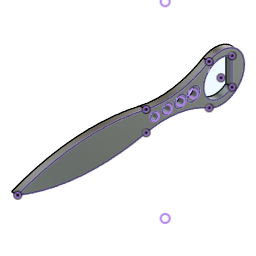
OpenBottleOpener (Autodesk Fusion 360 design; units mm, degrees)
Autodesk Fusion 360 part; units mm, degrees
sketch "Shape" plane through (0, 0, 0) normal (1, 0, 0) x (0, 1, 0)
  arc A0 (99.06, 7.7917) -> (0, 0) centre (62.0114, -154.7864) ccw
  arc A1 (99.06, 7.7917) -> (147.7109, 15.4666) centre (113.7922, 72.4404) ccw
  arc A2 (174.9187, 0) -> (147.7109, 15.4666) centre (156.9187, 0) ccw
  line L0 (0, 0) -> (174.9187, 0)
  arc A3 (170.4187, 0) -> (143.4187, 0) centre (156.9187, 0) ccw
  line L1 (165.4187, 10.4881) -> (165.4187, 0)
  circle A4 centre (115.4187, 0) radius 3.6667
  circle A5 centre (125.4187, 0) radius 4.3333
  circle A6 centre (135.4187, 0) radius 5
  circle A7 centre (105.4187, 0) radius 3
  line L2 (105.2187, -2.9933) -> (135.0854, -4.9889)
  line L3 (105.4187, 0) -> (115.4187, 0)
  line L4 (115.4187, 0) -> (125.4187, 0)
  line L5 (125.4187, 0) -> (135.4187, 0)
  line L6 (102.4187, 0) -> (0, 0)
  line L7 (140.4187, 0) -> (143.4187, 0)
  line L8 (170.4187, 0) -> (174.9187, 0)
  line L9 (170.4187, 0) -> (165.4187, 0)
  dimension "d2" = 99.06
  dimension "d3" = 18
  dimension "d10" = 174.9187
  dimension "d11" = 13.5
  dimension "d12" = 8.5
  dimension "d13" = 6
  dimension "d14" = 10
  dimension "d15" = 10
  dimension "d16" = 8
  constraint coincident A0.end L0.start
  constraint horizontal L0
  constraint tangent A0 A1
  constraint tangent A1 A2
  constraint horizontal A2.start A2.centre
  constraint coincident L0 A3.start
  constraint coincident A2.centre A3.centre
  constraint coincident L0 A3.end
  constraint coincident A3 L1.start
  constraint coincident L0 L1.end
  constraint perpendicular L0 L1
  constraint coincident L0 A4.centre
  constraint coincident L0 A5.centre
  constraint coincident L0 A6.centre
  constraint coincident L0 A7.centre
  constraint coincident A7 L2.start
  constraint coincident A6 L2.end
  constraint tangent A6 L2
  constraint tangent A7 L2
  constraint tangent A5 L2
  constraint tangent A4 L2
  constraint coincident A7.centre L3.start
  constraint coincident A4.centre L3.end
  constraint coincident A5.centre L4.end
  constraint coincident A6.centre L5.end
  constraint equal L3 L4
  constraint equal L4 L5
  constraint coincident A7 L6.start
  constraint coincident L0 L6.start
  constraint coincident A6 L7.start
  constraint coincident L0 L7.start
  measures "d2" horizontal distance of A0.end A0.start
  measures "d3" radius of A2
  measures "d10" distance of A0.end A2.start
  measures "d11" radius of A3
  measures "d12" distance of A2.centre L1
  measures "d13" diameter of A7
  measures "d14" diameter of A6
  measures "d15" distance of A4.centre A7.centre
  measures "d16" distance of A3.end A6.centre
extrude "Extrude1" add sketch "Shape" along normal blind 4.7498 contours A0 A1 A2 L0 A3 A4 A5 A6 A7 L3 L4 L5 L6 L7 L8 | L0 A3 L1 L9
mirror "Mirror1" about plane through (0, 0, 0) normal (0, 0, -1) of bodies 1 merged
sketch "DXF_export" plane through (4.7498, 0, 0) normal (1, 0, 0) x (0, 1, 0)
  arc A0 (165.4187, 10.4881) -> (165.4187, -10.4881) centre (156.9187, 0) ccw
  line L0 (165.4187, 10.4881) -> (165.4187, -10.4881)
  circle A1 centre (135.4187, 0) radius 5
  circle A2 centre (125.4187, 0) radius 4.3333
  circle A3 centre (115.4187, 0) radius 3.6667
  circle A4 centre (105.4187, 0) radius 3
  arc A5 (0, 0) -> (99.06, -7.7917) centre (62.0114, 154.7864) ccw
  arc A6 (147.7109, -15.4666) -> (99.06, -7.7917) centre (113.7922, -72.4404) ccw
  arc A7 (147.7109, -15.4666) -> (147.7109, 15.4666) centre (156.9187, 0) ccw
  arc A8 (99.06, 7.7917) -> (147.7109, 15.4666) centre (113.7922, 72.4404) ccw
  arc A9 (99.06, 7.7917) -> (0, 0) centre (62.0114, -154.7864) ccw
